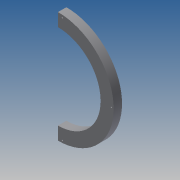
# Autodesk Inventor part: wheel_rim_mold_B_Prime
Saved by Autodesk Inventor 2014 SP2 (Build 180246200, 246)
## iProperties
Created: 2014-08-02
Part Number: wheel_rim_mold_B_Prime
Material: Générique
Document SubType Name: Modeling
Designer: Yann
Density: 1 g/cm^3
Appearance: Par défaut
Author: Yann
Autodesk Inventor part; units mm, degrees
ref_plane "YZ Plane" through (0, 0, 0) normal (1, 0, 0) x (0, 1, 0)
ref_plane "Plan de construction1" through (0, 20, -215.2) normal (0, 1, 0) x (0, 0, 1)
ref_plane "Plan de construction2" through (0, -20, -215.2) normal (0, -1, 0) x (1, 0, 0)
sketch "Esquisse1" plane through (0, 0, 0) normal (0, 1, 0) x (-1, 0, 0)
  circle A0 centre (0, 0) radius 203.2 construction
  circle A1 centre (-20, 253.412) radius 4
  circle A2 centre (-254.2, 0) radius 4
  circle A3 centre (-20, -253.412) radius 4
  line L0 (0, 215.2) -> (0, 265.412)
  line L1 (0, -265.412) -> (0, -215.2)
  line L2 (0, -410.2053) -> (0, 403.2318) construction
  line L3 (-446.5269, 0) -> (446.5269, 0) construction
  arc A4 (0, 265.412) -> (0, -265.412) centre (0, 0) ccw
  arc A5 (0, 203.2) -> (0, -203.2) centre (0, 0) ccw
  line L4 (0, 203.2) -> (0, 265.412)
  line L5 (0, -265.412) -> (0, -203.2)
  point P0 (0, 0)
extrude "Extrusion1" add sketch "Esquisse1" against normal up to surface (40 mm away) from surface at 20
sketch "Esquisse2" plane through (0, 20, 0) normal (0, 1, 0) x (1, 0, 0)
  line L0 (0, 215.2) -> (0, 265.412) construction
  arc A0 (0, -215.2) -> (0, 215.2) centre (0, 0) ccw projected
  line L1 (0, -265.412) -> (0, -215.2) construction
  arc A1 (0, -227.9) -> (0, 227.9) centre (0, 0) ccw
  arc A2 (0, -215.2) -> (0, 215.2) centre (0, 0) ccw projected
  line L2 (0, 215.2) -> (0, 227.9)
  line L3 (0, -227.9) -> (0, -215.2)
  dimension "d2" = 12.7
  constraints: 4 end point, 2 collinear, 2 point on circle, 1 centre point, 1 coincident, 1 point on line
  measures "d2" radial gap between concentric circles of A2 A1
extrude "Extrusion2" cut sketch "Esquisse2" against normal blind 3
